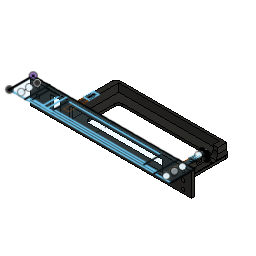
module_lanberg_dsp1-1008 (Autodesk Fusion 360 design; units mm, degrees)
Autodesk Fusion 360 part; units mm, degrees
sketch "Sketch1" plane through (0, 0, 0) normal (0, 0, 1) x (1, 0, 0)
  line L0 (0, 0) -> (200, 0) construction
  line L1 (200, 0) -> (200, -30)
  line L2 (200, -30) -> (0, -30) construction
  line L3 (0, -30) -> (0, 0)
  line L4 (0, 0) -> (0, -0.5) construction
  line L5 (0, -30) -> (0, -29.5) construction
  line L6 (0, -0.5) -> (200, -0.5)
  line L7 (200, -0.5) -> (200, -29.5)
  line L8 (200, -29.5) -> (0, -29.5)
  line L9 (0, -29.5) -> (0, -0.5)
  line L10 (0, 0) -> (20, 0) construction
  line L11 (20, 0) -> (20, -30)
  line L12 (20, -30) -> (0, -30) construction
  line L13 (0, -30) -> (0, 0) construction
  line L14 (200, 0) -> (180, 0) construction
  line L15 (180, 0) -> (180, -30)
  line L16 (180, -30) -> (200, -30) construction
  line L17 (200, -30) -> (200, 0) construction
  line L18 (100, 0) -> (100, -29.5) construction
  line L19 (10, 0) -> (10, -30) construction
  line L20 (10, 0) -> (10, -5) construction
  circle A0 centre (10, -5) radius 2.1
  circle A1 centre (10, -15) radius 2.1
  circle A2 centre (10, -25) radius 2.1
  circle A3 centre (190, -5) radius 2.1
  circle A4 centre (190, -15) radius 2.1
  circle A5 centre (190, -25) radius 2.1
  line L21 (180, -29.5) -> (20, -29.5) construction
  line L22 (20, -29.5) -> (20, -26.5) construction
  line L23 (20, -26.5) -> (180, -26.5)
  line L24 (180, -26.5) -> (180, -29.5) construction
  line L25 (180, -26.5) -> (164, -26.5)
  line L26 (49, -26.5) -> (38, -26.5)
  line L27 (38, -26.5) -> (38, -25.5)
  line L28 (20, 0) -> (20, -5)
  line L29 (20, -5) -> (25, -5)
  line L30 (38, -25.5) -> (25, -25.5)
  line L31 (25, -25.5) -> (25, -5)
  line L32 (25, -5) -> (38, -5)
  line L33 (38, -5) -> (38, -25.5)
  line L34 (164, -26.5) -> (164, -23.5)
  line L35 (164, -23.5) -> (49, -23.5)
  line L36 (49, -23.5) -> (49, -5.5)
  line L37 (49, -5.5) -> (164, -5.5)
  line L38 (164, -5.5) -> (164, -23.5)
  line L39 (49, -26.5) -> (43.5, -26.5)
  line L40 (43.5, -26.5) -> (43.5, 0)
  dimension "d1" = 200
  dimension "d2" = 30
  dimension "d3" = 0.5
  dimension "d4" = 0.5
  dimension "d5" = 200
  dimension "d6" = 20
  dimension "d7" = 20
  dimension "d8" = 30
  dimension "d10" = 4.2
  dimension "d13" = 0
  dimension "d14" = -20
  dimension "d15" = 160
  dimension "d16" = 3
  dimension "d17" = 16
  dimension "d18" = 115
  dimension "d20" = 11
  dimension "d21" = 1
  dimension "d22" = 5
  dimension "d23" = 5
  dimension "d24" = 3
  dimension "d25" = 115
  dimension "d26" = 18
  constraint horizontal L0
  constraint vertical L1
  constraint horizontal L2
  constraint vertical L3
  constraint coincident L0.start L3.end
  constraint perpendicular L0 L4
  constraint vertical L5
  constraint horizontal L6
  constraint vertical L7
  constraint horizontal L8
  constraint vertical L9
  constraint horizontal L10
  constraint vertical L11
  constraint horizontal L12
  constraint vertical L13
  constraint horizontal L14
  constraint vertical L15
  constraint horizontal L16
  constraint vertical L17
  constraint midpoint L0 L18.start
  constraint midpoint L8 L18.end
  constraint midpoint L10 L19.start
  constraint midpoint L12 L19.end
  constraint coincident L19 L20.end
  constraint coincident L20.end A0.centre
  constraint symmetric L18 A0 A3
  constraint symmetric L18 A1 A4
  constraint symmetric L18 A2 A5
  constraint horizontal L21
  constraint vertical L22
  constraint horizontal L23
  constraint vertical L24
  constraint coincident L8 L21.start
  constraint coincident L15 L21.start
  constraint perpendicular L15 L25
  constraint perpendicular L23 L27
  constraint perpendicular L0 L28
  constraint perpendicular L28 L29
  constraint horizontal L30
  constraint vertical L31
  constraint horizontal L32
  constraint vertical L33
  constraint perpendicular L23 L34
  constraint horizontal L35
  constraint vertical L36
  constraint horizontal L37
  constraint vertical L38
  constraint midpoint L26 L39.end
  constraint parallel L23 L39
  constraint coincident L0 L40.end
  constraint perpendicular L0 L40
  measures "d1" distance of L0.start L0.end
  measures "d2" distance of L0.start L2.end
  measures "d3" distance of L0.start L4.end
  measures "d4" distance of L2.end L5.end
  measures "d5" distance of L4.end L6.end
  measures "d6" distance of L0.start L10.end
  measures "d7" distance of L0.end L14.end
  measures "d8" distance of L0.end L1.end
  measures "d10" diameter of A0
  measures "d15" distance of L21.start L21.end
  measures "d16" distance of L21.start L23.end
  measures "d17" distance of L23.end L25.end
  measures "d18" distance of L25.end L26.start
  measures "d20" distance of L26.start L26.end
  measures "d21" distance of L26.end L27.end
  measures "d22" distance of L10.end L28.end
  measures "d23" distance of L28.end L29.end
  measures "d24" distance of L25.end L34.end
  measures "d25" distance of L34.end L35.end
  measures "d26" distance of L34.end L37.end
  measures "d77" distance of L0.start
extrude "Extrude1" add sketch "Sketch1" along normal blind 4 contours L1 L6 L7 L8 L15 | L6 L15 L23 L25 L26 L39 L40 | L8 L11 L15 L23 L25 L26 L39 | L6 L11 L23 L26 L27 L28 L29 L32 L33 L40 | L3 L6 L8 L9 L11 L28 | L11 L23 L27 L29 L30 L31 makes body 1
fillet "Fillet1" radius 2 4 edges at (25, -5, 2) (38, -5, 2) (38, -25.5, 2) (25, -25.5, 2) on bodies 1
fillet "Fillet2" radius 1 4 edges at (49, -23.5, 2) (49, -5.5, 2) (164, -5.5, 2) (164, -23.5, 2) on bodies 1
fillet "Fillet3" [suppressed]
fillet "Fillet4" [suppressed]
copy_body "Body->Comp1" bodies 1 removing the originals makes body 2 in component "lanberg_mount"
copy_body "Body->Comp1'" bodies 2 removing the originals makes body 3 in component "front"
extrude "Extrude1'" add sketch "Sketch1" against normal blind 65 contours L8 L11 L15 L23 L25 L26 L39 bodies 3 in component "front"
extrude "Extrude2" cut 1 faces at (180, -27.5, -21.6667) along direction (-1, 0, 0) blind 1 on bodies 3 bodies 3 in component "front"
extrude "Extrude3" cut 1 faces at (20, -27.5, -21.6667) along direction (1, 0, 0) blind 1 on bodies 3 bodies 3 in component "front"
sketch "Sketch3" plane through (0, -26.5, 0) normal (0, 1, 0) x (-1, 0, 0)
  line L0 (-21, -65) -> (-21, 0)
  line L1 (-21, 0) -> (-179, 0)
  line L2 (-179, 0) -> (-179, -65)
  line L3 (-179, -65) -> (-21, -65)
  line L4 (-164, 0) -> (-169, 0) construction
  line L5 (-169, 0) -> (-175, 0)
  line L6 (-169, 0) -> (-44, 0)
  line L7 (-44, 0) -> (-44, -62)
  line L8 (-44, -62) -> (-169, -62)
  line L9 (-169, -62) -> (-169, 0)
  line L10 (-169, -62) -> (-169, -54) construction
  line L11 (-169, -62) -> (-169, -40) construction
  line L12 (-175, 0) -> (-175, -65)
  line L13 (-169, -40) -> (-175, -40)
  line L14 (-175, -40) -> (-175, -54)
  line L15 (-175, -54) -> (-169, -54)
  line L16 (-169, -54) -> (-169, -40)
  line L17 (-44, -62) -> (-44, -65) construction
  line L18 (-44, -65) -> (-38, -65) construction
  line L19 (-38, -65) -> (-38, 0)
  dimension "d47" = 5
  dimension "d48" = 6
  dimension "d49" = 125
  dimension "d50" = 62
  dimension "d51" = 8
  dimension "d52" = 22
  dimension "d53" = 6
  constraint coincident L1 L4.start
  constraint parallel L1 L4
  constraint parallel L1 L5
  constraint horizontal L6
  constraint vertical L7
  constraint horizontal L8
  constraint vertical L9
  constraint perpendicular L8 L10
  constraint perpendicular L8 L11
  constraint coincident L3 L12.end
  constraint perpendicular L3 L12
  constraint horizontal L13
  constraint vertical L14
  constraint horizontal L15
  constraint vertical L16
  constraint coincident L12 L14.end
  constraint coincident L3 L17.end
  constraint perpendicular L8 L17
  constraint perpendicular L17 L18
  constraint coincident L1 L19.end
  constraint perpendicular L1 L19
  measures "d47" distance of L4.start L4.end
  measures "d48" distance of L4.end L5.end
  measures "d49" distance of L4.end L6.end
  measures "d50" distance of L4.end L8.end
  measures "d51" distance of L8.end L10.end
  measures "d52" distance of L8.end L11.end
  measures "d53" distance of L17.end L18.end
extrude "Extrude4" add sketch "Sketch3" along normal blind 10 contours L1 L3 L7 L8 L9 L12 L15 L19 | L1 L5 L9 L12 L13 bodies 3 in component "front"
fillet "Fillet1'" radius 5 2 edges at (172, -26.5, -40) (172, -26.5, -54) on bodies 3 in component "front"
sketch "Sketch4" plane through (0, 0, -16.5) normal (0, 0, 1) x (-1, 0, 0)
  line L0 (-169, 0) -> (-175, 0)
  line L1 (-175, 0) -> (-175, -40)
  line L2 (-175, -40) -> (-169, -40)
  line L3 (-169, -40) -> (-169, 0)
  line L4 (-175, 0) -> (-169, 0) construction
  line L5 (-169, 0) -> (-169, -25) construction
  line L6 (-169, -25) -> (-175, -25) construction
  line L7 (-175, -25) -> (-175, 0) construction
  line L8 (-44, 0) -> (-38, 0) construction
  line L9 (-38, 0) -> (-38, -25) construction
  line L10 (-38, -25) -> (-44, -25) construction
  line L11 (-44, -25) -> (-44, 0) construction
  line L12 (-44, -25) -> (-38, -25)
  line L13 (-38, -25) -> (-38, -37)
  line L14 (-38, -37) -> (-44, -37)
  line L15 (-44, -37) -> (-44, -25)
  line L16 (-175, -25) -> (-169, -25)
  line L17 (-169, -25) -> (-169, -37)
  line L18 (-169, -37) -> (-175, -37)
  line L19 (-175, -37) -> (-175, -25)
  line L20 (-169, -37) -> (-171, -37) construction
  line L21 (-171, -37) -> (-171, -25) construction
  line L22 (-171, -25) -> (-169, -25) construction
  line L23 (-169, -25) -> (-169, -37) construction
  line L24 (-171, -31) -> (-171, -34) construction
  line L25 (-171, -31) -> (-171, -28) construction
  line L26 (-171, -28) -> (-173, -28)
  line L27 (-173, -28) -> (-173, -34)
  line L28 (-173, -34) -> (-171, -34)
  line L29 (-171, -34) -> (-171, -28)
  dimension "d57" = 25
  dimension "d58" = 25
  dimension "d59" = 6
  dimension "d60" = 12
  dimension "d61" = 2
  dimension "d62" = 12
  dimension "d63" = 3
  dimension "d64" = 3
  dimension "d65" = 2
  constraint horizontal L4
  constraint vertical L5
  constraint horizontal L6
  constraint vertical L7
  constraint coincident L0.end L1.start
  constraint horizontal L8
  constraint vertical L9
  constraint horizontal L10
  constraint vertical L11
  constraint horizontal L12
  constraint vertical L13
  constraint horizontal L14
  constraint vertical L15
  constraint horizontal L16
  constraint vertical L17
  constraint horizontal L18
  constraint vertical L19
  constraint horizontal L20
  constraint vertical L21
  constraint horizontal L22
  constraint vertical L23
  constraint midpoint L21 L24.start
  constraint parallel L21 L24
  constraint parallel L21 L25
  constraint horizontal L26
  constraint vertical L27
  constraint horizontal L28
  constraint vertical L29
  measures "d57" distance of L0.end L6.end
  measures "d58" distance of L8.start L10.end
  measures "d59" distance of L10.end L9.end
  measures "d60" distance of L6.end L18.end
  measures "d61" distance of L17.end L20.end
  measures "d62" distance of L17.end L5.end
  measures "d63" distance of L24.start L24.end
  measures "d64" distance of L24.start L25.end
  measures "d65" distance of L25.end L26.end
sketch "Sketch5" plane through (0, 40, 0) normal (0, 1, 0) x (-1, 0, 0)
  line L0 (-175, -21.5) -> (-169, -21.5)
  line L1 (-169, -21.5) -> (-169, -16.5)
  line L2 (-169, -16.5) -> (-175, -16.5)
  line L3 (-175, -16.5) -> (-175, -21.5)
  line L4 (-169, -16.5) -> (-170, -16.5) construction
  line L5 (-170, -16.5) -> (-170, -21.5) construction
  line L6 (-170, -21.5) -> (-169, -21.5) construction
  line L7 (-169, -21.5) -> (-169, -16.5) construction
  line L8 (-170, -16.5) -> (-172.3466, -16.5) construction
  line L9 (-170, -16.5) -> (-175, -21.5)
  line L10 (-172.3466, -16.5) -> (-175, -19)
  dimension "d66" = 1
  constraint horizontal L4
  constraint vertical L5
  constraint horizontal L6
  constraint vertical L7
  constraint coincident L1.end L2.start
  constraint coincident L2 L8.end
  constraint perpendicular L5 L8
  constraint coincident L0.start L3.end
  constraint midpoint L3 L10.end
  measures "d66" distance of L1.end L4.end
extrude "Extrude2'" add sketch "Sketch5" along normal blind -6 and the other way blind 12 separate body contours L2 L3 L9 L10 makes body 4
ref_plane "WorkPlane1" through (106.5, 20, -21.5) normal (-1, 0, 0) x (0, -1, 0)
mirror "Mirror1" about plane through (106.5, 20, -21.5) normal (-1, 0, 0) of bodies 4 makes body 5
combine "Combine1" operation cut target body 3 tool bodies 4 5 body 4 seen with x (1, 0, 0) y (0, 0, -1) z (0, 1, 0) at (0, 0, 0) body 5 seen with x (1, 0, 0) y (0, 0, -1) z (0, 1, 0) at (0, 0, 0) keep tools in component "front"
copy_body "Body->Comp2" bodies 4 removing the originals makes body 6 in component "Cutter"
copy_body "CutPasteBodies1" bodies 5 removing the originals makes body 7 in component "Cutter"
fillet "Fillet2'" radius 3 2 edges at (175, -26.5, -57) (175, -26.5, -22.5) on bodies 3 in component "front"
fillet "Fillet3'" radius 15 2 edges at (172, -16.5, 0) (41, -16.5, 0) on bodies 3 in component "front"
sketch "Sketch6" plane through (0, 0, -26.5) normal (0, 0, 1) x (-1, 0, 0)
  line L0 (-38, 0) -> (-38, -65)
  line L1 (-38, -65) -> (-21, -65)
  line L2 (-21, -65) -> (-21, 0)
  line L3 (-21, 0) -> (-38, 0)
  line L4 (-38, -65) -> (-21, 0)
  constraint coincident L0.end L1.start
  constraint coincident L2.end L3.start
extrude "Extrude5" cut sketch "Sketch6" against normal blind 20 contours L1 L2 L4 sketch seen with x (1, 0, 0) y (0, 0, -1) z (0, 1, 0) at (0, 0, 0) bodies 3 in component "front"
sketch "Sketch7" plane through (0, 0, -16.5) normal (0, 0, 1) x (-1, 0, 0)
  line L0 (-169, -15) -> (-175, -15)
  line L1 (-175, -15) -> (-175, -40)
  line L2 (-175, -40) -> (-169, -40)
  line L3 (-169, -40) -> (-169, -15)
  line L4 (-170, -34) -> (-172.3466, -34)
  line L5 (-172.3466, -34) -> (-172.3466, -28)
  line L6 (-172.3466, -28) -> (-170, -28)
  line L7 (-170, -28) -> (-170, -34)
  line L8 (-175, -40) -> (-172.3466, -40)
  line L9 (-172.3466, -40) -> (-172.3466, -22)
  line L10 (-172.3466, -22) -> (-175, -22)
  line L11 (-175, -22) -> (-175, -40)
  dimension "d77" = 18
  constraint horizontal L8
  constraint vertical L9
  constraint horizontal L10
  constraint vertical L11
  constraint coincident L1.end L2.start
  measures "d77" distance of L1.end L10.end
sketch "Sketch8" plane through (0, 0, -26.5) normal (0, 0, 1) x (-1, 0, 0)
  line L0 (-178, -45) -> (-178, 0)
  line L1 (-178, 0) -> (-179, 0)
  line L2 (-179, 0) -> (-179, -65)
  line L3 (-179, -65) -> (-178, -65)
  line L4 (-178, -65) -> (-178, -49)
  line L5 (-178, -49) -> (-169, -49)
  line L6 (-169, -49) -> (-169, -62)
  line L7 (-169, -62) -> (-44, -62)
  line L8 (-44, -62) -> (-44, 0)
  line L9 (-44, 0) -> (-169, 0)
  line L10 (-169, 0) -> (-169, -45)
  line L11 (-169, -45) -> (-178, -45)
  line L12 (-44, 0) -> (-169, 0) construction
  line L13 (-169, 0) -> (-169, -62) construction
  line L14 (-169, -62) -> (-44, -62) construction
  line L15 (-44, -62) -> (-44, 0) construction
  line L16 (-54, -10) -> (-159, -10)
  line L17 (-159, -10) -> (-159, -52)
  line L18 (-159, -52) -> (-54, -52)
  line L19 (-54, -52) -> (-54, -10)
  dimension "d78" = -10
  constraint horizontal L12
  constraint vertical L13
  constraint horizontal L14
  constraint vertical L15
  constraint coincident L6.end L7.start
  constraint coincident L8.end L9.start
extrude "Extrude6" cut sketch "Sketch8" against normal blind 100 contours L16 L17 L18 L19 sketch seen with x (1, 0, 0) y (0, 0, -1) z (0, 1, 0) at (0, 0, 0) bodies 3 in component "front"
fillet "Fillet4'" radius 5 4 edges at (159, -28, -10) (54, -28, -10) (54, -28, -52) (159, -28, -52) on bodies 3 in component "front"
fillet "Fillet5" radius 5 1 edges at (179, -28, -65) on bodies 3 in component "front"
fillet "Fillet6" radius 5 2 edges at (38, -21.5, -65) (38, -28, -65) on bodies 3 in component "front"
component "lanberg_mount" placed x (1, 0, 0) y (0, 0, 1) z (0, -1, 0) at (0, 0, 0)
component "Cutter" placed x (1, 0, 0) y (0, 1, 0) z (0, 0, 1) at (0, 0, 0)
component "front" placed x (1, 0, 0) y (0, 1, 0) z (0, 0, 1) at (0, 0, 0) in component "lanberg_mount"
equation "d17 = 5 mm + ridge_width + 5 mm"
equation "d18 = 125 mm - ( 5 * 2 ) * 1 mm"
equation "d20 = 5 mm + ridge_width"
equation "d25 = 125 mm - ( 5 * 2 ) * 1 mm"
equation "d33 = -62 mm - 3 mm"
equation "ridge_width = 6 mm"
equation "d48 = ridge_width"
equation "d53 = ridge_width"
equation "d71 = ( 125 / 2 ) * 1 mm"
equation "d77 = 15 mm + 3 mm"
